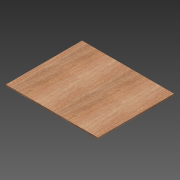
# Autodesk Inventor part: top_cover_sheet
Saved by Autodesk Inventor 2014 SP1 (Build 180222100, 222)
## iProperties
Created: 2014-02-23
Part Number: top_cover_sheet
Material: Wood (Birch)
Document SubType Name: Modeling
Designer: Chris
Density: 0.55 g/cm^3
Appearance: Birch - Natural Polished
Mass: 1233.22 g
Surface Area: 4893.74 cm^2
Volume: 2242.21 cm^3
Author: Chris
Autodesk Inventor part; units mm, degrees
ref_plane "YZ Plane" through (0, 0, 0) normal (1, 0, 0) x (0, 1, 0)
ref_plane "XZ Plane" through (0, 0, 0) normal (0, 1, 0) x (-1, 0, 0)
ref_plane "XY Plane" through (0, 0, 0) normal (0, 0, 1) x (1, 0, 0)
sketch "Sketch1" plane through (0, 0, 0) normal (0, 0, 1) x (1, 0, 0)
  line L0 (0, 0) -> (533.4, 0)
  line L1 (533.4, 0) -> (533.4, 9.525)
  line L2 (533.4, 9.525) -> (0, 9.525)
  line L3 (0, 9.525) -> (0, 0)
  dimension "d0" = 533.4
  dimension "d1" = 9.525
  constraints: 8 end point, 2 parallel, 1 horizontal, 1 perpendicular
  measures "d0" distance of L1.end L2.end
  measures "d1" distance of L0.end L1.end
extrude "Extrusion1" add sketch "Sketch1" along normal blind 441.325
body "Solid1"
